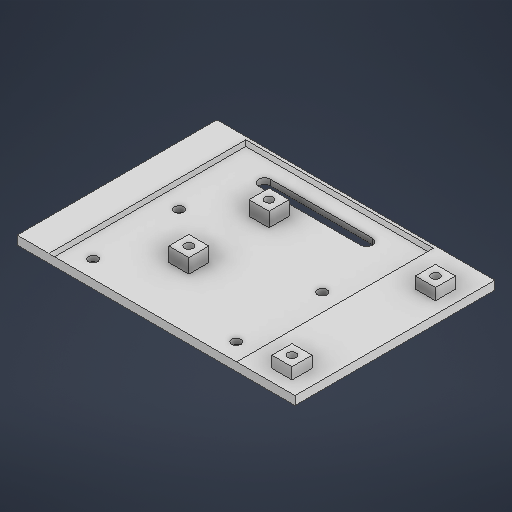
# Autodesk Inventor part: TOPLeft
Saved by Autodesk Inventor 2026.1 (Build 301233020, 233B)
## iProperties
Created: 2026-07-07
Part Number: TOPLeft
Material: Generic
Document SubType Name: Modeling
Designer: pleased
Density: 1 g/cm^3
Appearance: Default
Author: pleased
Autodesk Inventor part; units mm, degrees
ref_plane "YZ Plane" through (0, 0, 0) normal (1, 0, 0) x (0, 1, 0)
ref_plane "XZ Plane" through (0, 0, 0) normal (0, 1, 0) x (-1, 0, 0)
ref_plane "XY Plane" through (0, 0, 0) normal (0, 0, 1) x (1, 0, 0)
sketch "Sketch1" plane through (0, 0, 0) normal (0, 1, 0) x (-1, 0, 0)
  line L0 (0, 80) -> (150, 80)
  line L1 (150, 80) -> (150, 0)
  line L2 (150, 0) -> (0, 0)
  line L3 (0, 0) -> (0, 80)
  point P0 (0, 0)
  dimension "d0" = 150
  dimension "d1" = 80
  constraints: 8 end point, 2 parallel, 1 horizontal, 1 perpendicular
  measures "d0" distance of L1.end L2.end
  measures "d1" distance of L0.end L1.end
extrude "Extrusion1" add sketch "Sketch1" along normal blind 3
sketch "Sketch2" plane through (0, 3, 0) normal (0, 1, 0) x (1, 0, 0)
  line L0 (-93.7, -18) -> (-58, -18)
  line L1 (-93.7, -18) -> (-58, -18) construction
  line L2 (-93.7, -20.1) -> (-58, -20.1)
  line L3 (-58, -15.9) -> (-93.7, -15.9)
  arc A0 (-93.7, -15.9) -> (-93.7, -20.1) centre (-93.7, -18) ccw
  arc A1 (-58, -20.1) -> (-58, -15.9) centre (-58, -18) ccw
  circle A2 centre (-100.5, -71) radius 1.65
  circle A3 centre (-100.5, -41) radius 1.65
  circle A4 centre (-50.5, -71) radius 1.65
  circle A5 centre (-50.5, -41) radius 1.65
  point P0 (0, 0)
  point P1 (-50.5, -18)
  point P2 (-92, -41)
  point P3 (-92, -71)
  point P4 (-75.85, -18)
  dimension "d4" = 4.2
  dimension "d5" = 3.3
  dimension "d6" = 3.3
  dimension "d7" = 3.3
  dimension "d8" = 3.3
  constraints: 10 end point, 6 centre point, 4 coincident, 4 point on circle, 4 tangent, 2 equal length, 1 horizontal, 1 midpoint
  measures "d4" diameter of A1
  measures "d5" diameter of A2
  measures "d6" diameter of A3
  measures "d7" diameter of A4
  measures "d8" diameter of A5
extrude "Extrusion2" cut sketch "Sketch2" against normal blind 3
sketch "Sketch3" plane through (0, 3, 0) normal (0, 1, 0) x (1, 0, 0)
  line L0 (-107.9014, -77.0296) -> (-44.3595, -77.0296)
  line L1 (-44.3595, -77.0296) -> (-44.3595, -10.2906)
  line L2 (-44.3595, -10.2906) -> (-107.9014, -10.2906)
  line L3 (-107.9014, -10.2906) -> (-107.9014, -77.0296)
  point P0 (0, 0)
  constraints: 8 end point, 2 parallel, 1 horizontal, 1 perpendicular
extrude "Extrusion3" cut sketch "Sketch3" against normal blind 1
chamfer "Chamfer1" distance 1 angle 45 4 edges at (-107.9014, 3, 43.6601) (-76.1304, 3, 10.2906) (-44.3595, 3, 43.6601) (-76.1304, 3, 77.0296)
sketch "Sketch4" plane through (0, 3, 0) normal (0, 1, 0) x (1, 0, 0)
  line L0 (-83.7407, -25.8238) -> (-30.7407, -25.8238)
  line L1 (-30.639, -72.8238) -> (-31.7407, -72.8238)
  line L2 (-31.7407, -70.3238) -> (-30.7407, -70.3238)
  line L3 (-30.639, -70.3238) -> (-30.639, -72.8238)
  line L4 (-27.139, -17.8238) -> (-34.139, -17.8238)
  line L5 (-34.139, -17.8238) -> (-34.139, -24.8238)
  line L6 (-34.139, -24.8238) -> (-27.139, -24.8238)
  line L7 (-27.139, -24.8238) -> (-27.139, -17.8238)
  line L8 (-27.139, -17.8238) -> (-34.139, -24.8238) construction
  line L9 (-34.139, -17.8238) -> (-27.139, -24.8238) construction
  line L10 (-28.2407, -73.8238) -> (-35.2407, -73.8238)
  line L11 (-35.2407, -73.8238) -> (-35.2407, -66.8238)
  line L12 (-35.2407, -66.8238) -> (-28.2407, -66.8238)
  line L13 (-28.2407, -66.8238) -> (-28.2407, -73.8238)
  line L14 (-28.2407, -73.8238) -> (-35.2407, -66.8238) construction
  line L15 (-35.2407, -73.8238) -> (-28.2407, -66.8238) construction
  line L16 (-30.639, -24.8238) -> (-82.7407, -24.8238)
  line L17 (-30.639, -58.4962) -> (-30.639, -24.8238)
  line L18 (-82.639, -58.4962) -> (-82.7407, -72.8238)
  line L19 (-82.7407, -72.8238) -> (-82.7407, -56.8238)
  line L20 (-82.7407, -56.8238) -> (-82.7407, -55.3238)
  line L21 (-79.2407, -58.8238) -> (-86.2407, -58.8238)
  line L22 (-86.2407, -58.8238) -> (-86.2407, -51.8238)
  line L23 (-86.2407, -51.8238) -> (-79.2407, -51.8238)
  line L24 (-79.2407, -51.8238) -> (-79.2407, -58.8238)
  line L25 (-79.2407, -58.8238) -> (-86.2407, -51.8238) construction
  line L26 (-86.2407, -58.8238) -> (-79.2407, -51.8238) construction
  line L27 (-82.7407, -55.3238) -> (-82.7407, -27.3238)
  line L28 (-79.2407, -30.8238) -> (-86.2407, -30.8238)
  line L29 (-86.2407, -30.8238) -> (-86.2407, -23.8238)
  line L30 (-86.2407, -23.8238) -> (-79.2407, -23.8238)
  line L31 (-79.2407, -23.8238) -> (-79.2407, -30.8238)
  line L32 (-79.2407, -30.8238) -> (-86.2407, -23.8238) construction
  line L33 (-86.2407, -30.8238) -> (-79.2407, -23.8238) construction
  point P0 (0, 0)
  constraints: 68 end point
extrude "Extrusion4" add sketch "Sketch4" along normal blind 4 and the other way blind 2 contours L7 L6 L5 L4 | L10 L11 L12 L13 | L21 L19 L20 L27 L23 L24 | L21 L22 L23 L27 L20 L19 | L28 L29 L30 L31
sketch "Sketch6" plane through (0, 7, 0) normal (0, 1, 0) x (1, 0, 0)
  line L0 (-86.2407, -51.8238) -> (-79.2407, -51.8238) projected
  line L1 (-79.2407, -51.8238) -> (-79.2407, -58.8238) projected
  line L2 (-86.2407, -51.8238) -> (-79.2407, -58.8238)
  line L3 (-86.2407, -30.8238) -> (-86.2407, -23.8238) projected
  line L4 (-86.2407, -30.8238) -> (-79.2407, -30.8238) projected
  line L5 (-86.2407, -23.8238) -> (-79.2407, -30.8238)
  line L6 (-34.139, -17.8238) -> (-27.139, -17.8238) projected
  line L7 (-27.139, -17.8238) -> (-27.139, -24.8238) projected
  line L8 (-34.139, -17.8238) -> (-27.139, -24.8238)
  line L9 (-35.2407, -73.8238) -> (-35.2407, -66.8238) projected
  line L10 (-28.2407, -73.8238) -> (-28.2407, -66.8238) projected
  line L11 (-35.2407, -66.8238) -> (-28.2407, -73.8238)
  circle A0 centre (-82.7407, -55.3238) radius 1.5
  circle A1 centre (-82.7407, -27.3238) radius 1.5
  circle A2 centre (-30.639, -21.3238) radius 1.5
  circle A3 centre (-31.7407, -70.3238) radius 1.5
  point P0 (0, 0)
  point P1 (-123.6624, -66.5994)
  point P2 (-116.6624, -73.5994)
  point P3 (-117.764, -24.5994)
  point P4 (-117.764, -17.5994)
  point P5 (-124.764, -17.5994)
  point P6 (-72.6624, -51.5994)
  dimension "d45" = 3
  dimension "d46" = 3
  dimension "d47" = 3
  dimension "d48" = 3
  constraints: 8 end point, 4 centre point, 4 midpoint
  measures "d45" diameter of A0
  measures "d46" diameter of A1
  measures "d47" diameter of A2
  measures "d48" diameter of A3
extrude "Extrusion5" cut sketch "Sketch6" against normal blind 4 contours A0 L2 | L2 A0 | A1 L5 | L5 A1 | A2 L8 | L8 A2 | A3 L11 | L11 A3
move faces "Move1" translate (-23, 0, 0) faces at (0, 1, 53.3333)
move faces "Move2" translate (0, 0, 8.25) faces at (-65.3333, 1, 0)
move faces "Move3" translate (0, 0, -2) faces at (-107.6667, 2, 80)
move faces "Move4" translate (30, 0, 0) faces at (-150, 1, 31.5)
body "Solid1"
